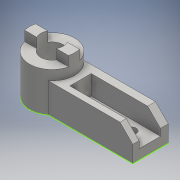
# Autodesk Inventor part: 240510_3Dsketch06
Saved by Autodesk Inventor 2016 (Build 200138000, 138)
## iProperties
Created: 2024-05-10
Part Number: 240510_3Dsketch06
Material: 일반
Document SubType Name: Modeling
Designer: pc
Density: 1 g/cm^3
Appearance: 기본값
Author: pc
Autodesk Inventor part; units mm, degrees
ref_plane "YZ Plane" through (0, 0, 0) normal (1, 0, 0) x (0, 1, 0)
ref_plane "XZ Plane" through (0, 0, 0) normal (0, 1, 0) x (-1, 0, 0)
ref_plane "XY Plane" through (0, 0, 0) normal (0, 0, 1) x (1, 0, 0)
sketch "스케치1" plane through (0, 0, 0) normal (0, 0, 1) x (1, 0, 0)
  circle A0 centre (-35.1217, 0) radius 22.9499
  circle A1 centre (-35.1217, 0) radius 11.4294
  line L0 (-20.9226, -18.03) -> (64.9173, -18.03)
  line L1 (64.9173, -18.03) -> (64.9173, 18.03)
  line L2 (64.9173, 18.03) -> (-20.9226, 18.03)
  point P0 (0, 0)
  constraints: 6 end point, 2 centre point, 2 perpendicular, 2 point on circle, 1 coincident, 1 horizontal
extrude "돌출1" add sketch "스케치1" along normal blind 30 contours A0 L2 L1 L0
extrude "돌출2" add sketch "스케치1" along normal blind 40 contours A0
sketch "스케치2" plane through (-35.1217, 0, 40) normal (0, 0, 1) x (1, 0, 0)
  circle A0 centre (0, 0) radius 11.4294 projected
  line L0 (9.9823, 5.5664) -> (22.2646, 5.5664)
  circle A1 centre (0, 0) radius 22.9499 projected
  line L1 (9.9823, -5.5664) -> (22.2646, -5.5664)
  line L2 (-9.9823, 5.5664) -> (-22.2646, 5.5664)
  line L3 (-9.9823, -5.5664) -> (-22.2646, -5.5664)
  point P0 (35.1217, 0)
  constraints: 8 end point, 8 point on circle, 4 point on line, 1 horizontal, 1 parallel
extrude "돌출3" add sketch "스케치2" along normal blind 10 contours A0 L0 A1 L1 | A0 L3 A1 L2
sketch "스케치3" plane through (0, 0, 30) normal (0, 0, 1) x (1, 0, 0)
  line L0 (64.9173, -18.03) -> (64.9173, 18.03) projected
  line L1 (-5.4969, 10.1103) -> (64.9173, 10.1103)
  line L2 (64.9173, 10.1103) -> (64.9173, -11.6809)
  line L3 (64.9173, -11.6809) -> (-5.4969, -11.6809)
  line L4 (-5.4969, -11.6809) -> (-5.4969, 10.1103)
  circle A0 centre (15.1164, 0) radius 4.8497
  circle A1 centre (45.3492, 0) radius 4.9674
  point P0 (0, 0)
  constraints: 8 end point, 2 centre point, 2 parallel, 1 horizontal, 1 perpendicular, 1 point on line
extrude "돌출4" cut sketch "스케치3" against normal blind 50 contours A0 | A1
extrude "돌출5" cut sketch "스케치3" against normal blind 20
chamfer "모따기1" distance 13 angle 45 2 edges at (64.9173, 14.0702, 30) (64.9173, -14.8554, 30)
